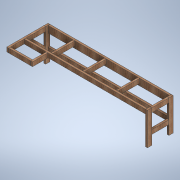
# Autodesk Inventor part: Frame Single
Saved by Autodesk Inventor 2020.2 (Build 242310000, 310)
## iProperties
Created: 2019-12-30
Part Number: Frame Single
Material: Wood (Birch - Stained)
Document SubType Name: Modeling
Designer: Andrew
Density: 0.1 g/cm^3
Appearance: Birch - Stained
Author: Andrew
Autodesk Inventor part; units mm, degrees
ref_plane "YZ Plane" through (0, 0, 0) normal (1, 0, 0) x (0, 1, 0)
ref_plane "XZ Plane" through (0, 0, 0) normal (0, 1, 0) x (-1, 0, 0)
ref_plane "XY Plane" through (0, 0, 0) normal (0, 0, 1) x (1, 0, 0)
derived "Desk Top Primary.ipt"
sketch "Primary Top" plane through (0, 0, 0) normal (0, 1, 0) x (-1, 0, 0)
  line L0 (-2713.228, 0) -> (-579.628, 0)
  line L1 (-579.628, 0) -> (-579.628, 143.3195)
  line L2 (-579.628, 143.3195) -> (-2713.228, 143.3195)
  line L3 (-2713.228, 143.3195) -> (-2713.228, 0)
  line L4 (-2713.228, 144.907) -> (-579.628, 144.907)
  line L5 (-579.628, 144.907) -> (-579.628, 288.2265)
  line L6 (-579.628, 288.2265) -> (-2713.228, 288.2265)
  line L7 (-2713.228, 288.2265) -> (-2713.228, 144.907)
  line L8 (-2713.228, 289.814) -> (-579.628, 289.814)
  line L9 (-579.628, 289.814) -> (-579.628, 433.1335)
  line L10 (-579.628, 433.1335) -> (-2713.228, 433.1335)
  line L11 (-2713.228, 433.1335) -> (-2713.228, 289.814)
  line L12 (-2713.228, 434.721) -> (-579.628, 434.721)
  line L13 (-579.628, 434.721) -> (-579.628, 578.0405)
  line L14 (-579.628, 578.0405) -> (-2713.228, 578.0405)
  line L15 (-2713.228, 578.0405) -> (-2713.228, 434.721)
  point P0 (0, 0)
derived "Desk Top Secondary.ipt"
sketch "Secondary Top" plane through (0, 0, 0) normal (0, 1, 0) x (-1, 0, 0)
  line L0 (0, 1270) -> (-143.3195, 1270)
  line L1 (-143.3195, 1270) -> (-143.3195, 0)
  line L2 (-143.3195, 0) -> (0, 0)
  line L3 (0, 0) -> (0, 1270)
  line L4 (-144.907, 1270) -> (-288.2265, 1270)
  line L5 (-288.2265, 1270) -> (-288.2265, 0)
  line L6 (-288.2265, 0) -> (-144.907, 0)
  line L7 (-144.907, 0) -> (-144.907, 1270)
  line L8 (-289.814, 1270) -> (-433.1335, 1270)
  line L9 (-433.1335, 1270) -> (-433.1335, 0)
  line L10 (-433.1335, 0) -> (-289.814, 0)
  line L11 (-289.814, 0) -> (-289.814, 1270)
  line L12 (-434.721, 1270) -> (-578.0405, 1270)
  line L13 (-578.0405, 1270) -> (-578.0405, 0)
  line L14 (-578.0405, 0) -> (-434.721, 0)
  line L15 (-434.721, 0) -> (-434.721, 1270)
sketch "Sketch3" plane through (0, 0, 0) normal (0, 1, 0) x (-1, 0, 0)
  line L0 (-12.7, 898.525) -> (-52.3966, 898.525)
  line L1 (-52.3966, 898.525) -> (-52.3966, 105.3465)
  line L2 (-52.3966, 105.3465) -> (-12.7, 105.3465)
  line L3 (-12.7, 105.3465) -> (-12.7, 898.525)
  line L4 (-12.7, 103.759) -> (-52.3966, 103.759)
  line L5 (-52.3966, 103.759) -> (-52.3966, 12.7)
  line L6 (-52.3966, 12.7) -> (-12.7, 12.7)
  line L7 (-12.7, 12.7) -> (-12.7, 103.759)
  line L8 (-53.9841, 12.7) -> (-2659.2439, 12.7)
  line L9 (-2659.2439, 12.7) -> (-2659.2439, 52.3966)
  line L10 (-2659.2439, 52.3966) -> (-53.9841, 52.3966)
  line L11 (-53.9841, 52.3966) -> (-53.9841, 12.7)
  line L12 (-2700.528, 12.7) -> (-2660.8314, 12.7)
  line L13 (-2660.8314, 12.7) -> (-2660.8314, 103.759)
  line L14 (-2660.8314, 103.759) -> (-2700.528, 103.759)
  line L15 (-2700.528, 103.759) -> (-2700.528, 12.7)
  line L16 (-2700.528, 105.3465) -> (-2660.8314, 105.3465)
  line L17 (-2660.8314, 105.3465) -> (-2660.8314, 472.694)
  line L18 (-2660.8314, 472.694) -> (-2700.528, 472.694)
  line L19 (-2700.528, 472.694) -> (-2700.528, 105.3465)
  line L20 (-2700.528, 474.2815) -> (-2660.8314, 474.2815)
  line L21 (-2660.8314, 474.2815) -> (-2660.8314, 565.3405)
  line L22 (-2660.8314, 565.3405) -> (-2700.528, 565.3405)
  line L23 (-2700.528, 565.3405) -> (-2700.528, 474.2815)
  line L24 (-2659.2439, 565.3405) -> (-53.9841, 565.3405)
  line L25 (-53.9841, 565.3405) -> (-53.9841, 525.6439)
  line L26 (-53.9841, 525.6439) -> (-2659.2439, 525.6439)
  line L27 (-2659.2439, 525.6439) -> (-2659.2439, 565.3405)
  line L28 (-53.9841, 898.525) -> (-524.0564, 898.525)
  line L29 (-524.0564, 898.525) -> (-524.0564, 858.8284)
  line L30 (-524.0564, 858.8284) -> (-53.9841, 858.8284)
  line L31 (-53.9841, 858.8284) -> (-53.9841, 898.525)
  line L32 (-565.3405, 898.525) -> (-525.6439, 898.525)
  line L33 (-525.6439, 898.525) -> (-525.6439, 566.928)
  line L34 (-525.6439, 566.928) -> (-565.3405, 566.928)
  line L35 (-565.3405, 566.928) -> (-565.3405, 898.525)
  line L36 (-2025.8314, 524.0564) -> (-1986.1349, 524.0564)
  line L37 (-1986.1349, 524.0564) -> (-1986.1349, 53.9841)
  line L38 (-1986.1349, 53.9841) -> (-2025.8314, 53.9841)
  line L39 (-2025.8314, 53.9841) -> (-2025.8314, 524.0564)
  line L40 (-592.328, 524.0564) -> (-632.0246, 524.0564)
  line L41 (-632.0246, 524.0564) -> (-632.0246, 53.9841)
  line L42 (-632.0246, 53.9841) -> (-592.328, 53.9841)
  line L43 (-592.328, 53.9841) -> (-592.328, 524.0564)
  line L44 (-1267.0246, 524.0564) -> (-1306.7211, 524.0564)
  line L45 (-1306.7211, 524.0564) -> (-1306.7211, 53.9841)
  line L46 (-1306.7211, 53.9841) -> (-1267.0246, 53.9841)
  line L47 (-1267.0246, 53.9841) -> (-1267.0246, 524.0564)
  point P0 (0, 0)
  point P1 (-2713.228, 578.0405)
  point P2 (-578.0405, 1270)
  point P3 (-579.628, 0)
  dimension "d2" = 39.6966
  dimension "d3" = 39.6966
  dimension "d4" = 39.6966
  dimension "d5" = 91.059
  dimension "d6" = 39.6966
  dimension "d7" = 39.6966
  dimension "d8" = 39.6966
  dimension "d10" = 39.6966
  dimension "d11" = 39.6966
  dimension "d12" = 91.059
  dimension "d13" = 91.059
  dimension "d14" = 39.6966
  dimension "d15" = 12.7
  dimension "d16" = 12.7
  dimension "d17" = 1.5875
  dimension "d18" = 1.5875
  dimension "d19" = 1.5875
  dimension "d20" = 1.5875
  dimension "d21" = 1.5875
  dimension "d22" = 1.5875
  dimension "d23" = 12.7
  dimension "d24" = 12.7
  dimension "d25" = 1.5875
  dimension "d26" = 1.5875
  dimension "d27" = 1.5875
  dimension "d28" = 1.5875
  dimension "d29" = 1.5875
  dimension "d30" = 1.5875
  dimension "d31" = 12.7
  dimension "d32" = 635
  dimension "d33" = 635
  dimension "d34" = 12.7
  dimension "d35" = 371.475
  dimension "d47" = 39.6966
  constraints: 96 end point, 24 parallel, 12 horizontal, 12 perpendicular, 11 point on line, 1 collinear
  measures "d2" distance of L0.start L0.end
  measures "d3" distance of L30.end L28.start
  measures "d4" distance of L32.start L32.end
  measures "d5" distance of L6.end L4.start
  measures "d6" distance of L24.end L25.end
  measures "d7" distance of L41.end L42.end
  measures "d8" distance of L45.end L46.end
  measures "d10" distance of L37.end L38.end
  measures "d11" distance of L12.start L12.end
  measures "d12" distance of L14.end L12.start
  measures "d13" distance of L22.end L20.start
  measures "d14" distance of L5.end L6.end
  measures "d15" horizontal distance of point (-2713.228, 578.041) L22.end
  measures "d16" horizontal distance of point (-2713.228, 578.041) L22.end
  measures "d17" distance between parallel lines of L21 L27
  measures "d18" distance between parallel lines of L18 L20
  measures "d19" distance between parallel lines of L14 L16
  measures "d20" distance between parallel lines of L13 L9
  measures "d21" distance between parallel lines of L11 L5
  measures "d22" distance between parallel lines of L2 L4
  measures "d23" horizontal distance of L6.end point (0, 0)
  measures "d24" horizontal distance of L6.end point (0, 0)
  measures "d25" distance between parallel lines of L10 L42
  measures "d26" distance between parallel lines of L26 L40
  measures "d27" distance between parallel lines of L24 L34
  measures "d28" distance between parallel lines of L33 L29
  measures "d29" distance between parallel lines of L31 L1
  measures "d30" distance between parallel lines of L25 L1
  measures "d31" horizontal distance of point (-578.041, 1270) L32.start
  measures "d32" distance between parallel lines of L47 L41
  measures "d33" distance between parallel lines of L17 L39
  measures "d34" distance from line of L43 point (-579.628, 0)
  measures "d35" vertical distance of point (-578.041, 1270) L32.start
  measures "d47" distance of L10.end L8.start
derived "Desk Drawer.ipt"
extrude "Extrusion1" add sketch "Sketch3" against normal blind 91.059 contours L3 L2 L1 L0 | L19 L18 L17 L16 | L24 L25 L26 L27 | L31 L30 L29 L28 | L32 L33 L34 L35 | L36 L37 L38 L39 | L43 L42 L41 L40 | L47 L46 L45 L44
extrude "Extrusion2" add sketch "Sketch3" against normal blind 698.5 contours L7 L6 L5 L4 | L15 L14 L13 L12 | L23 L22 L21 L20
derived "Frame Primary.ipt"
ref_plane "Support Plane" through (0, -495.3, 0) normal (0, 1, 0) x (-1, 0, 0)
extrude "Extrusion3" add sketch "Sketch3" along normal blind 91.059 from surface at -495.3 contours L8 L9 L10 L11 | L19 L18 L17 L16
extrude "Extrusion4" add sketch "Sketch3" against normal blind 143.3195 contours L8 L9 L10 L11
sketch "Sketch4" plane through (12.7, 0, 12.7) normal (-1, 0, 0) x (0, 0, 1)
  line L0 (366.5231, -92.6465) -> (92.6465, -366.5231)
  line L1 (92.6465, -366.5231) -> (92.6465, -495.3)
  line L2 (92.6465, -495.3) -> (495.3, -92.6465)
  line L3 (495.3, -92.6465) -> (366.5231, -92.6465)
  line L4 (91.059, 0) -> (91.059, -698.5) projected
  line L5 (885.825, -91.059) -> (92.6465, -91.059) projected
  point P0 (-12.7, 0)
  dimension "d48" = 1.5875
  dimension "d49" = 1.5875
  dimension "d50" = 91.059
  dimension "d51" = 45
  dimension "d52" = 203.2
  constraints: 8 end point, 1 parallel, 1 perpendicular, 1 vertical
  measures "d48" distance between parallel lines of L4 L1
  measures "d49" distance between parallel lines of L3 L5
  measures "d50" distance between parallel lines of L2 L0
  measures "d51" angle of L4 L0
  measures "d52" vertical distance of L4.end L1.end
extrude "Extrusion5" add sketch "Sketch4" against normal blind 39.6966
equation "\"d2\" = h_2x4"
equation "\"d3\" = h_2x4"
equation "\"d4\" = h_2x4"
equation "\"d5\" = w_2x4"
equation "\"d6\" = h_2x4"
equation "\"d7\" = h_2x4"
equation "\"d8\" = h_2x4"
equation "\"d10\" = h_2x4"
equation "\"d11\" = h_2x4"
equation "\"d12\" = w_2x4"
equation "\"d13\" = w_2x4"
equation "\"d14\" = h_2x4"
equation "\"d16\" = d15"
equation "\"d17\" = plank_tol"
equation "\"d18\" = plank_tol"
equation "\"d19\" = plank_tol"
equation "\"d20\" = plank_tol"
equation "\"d21\" = plank_tol"
equation "\"d22\" = plank_tol"
equation "\"d23\" = d15"
equation "\"d24\" = d15"
equation "\"d25\" = plank_tol"
equation "\"d26\" = plank_tol"
equation "\"d27\" = plank_tol"
equation "\"d28\" = plank_tol"
equation "\"d29\" = plank_tol"
equation "\"d30\" = plank_tol"
equation "\"d31\" = d15"
equation "\"d34\" = d15"
equation "\"d47\" = h_2x4"
equation "\"d37\" = w_2x4"
equation "\"d39\" = drawer_height"
equation "\"d42\" = w_2x4"
equation "\"d45\" = w_2x6"
equation "\"d48\" = plank_tol"
equation "\"d49\" = plank_tol"
equation "\"d50\" = w_2x4"
equation "\"d53\" = h_2x4"
equation "\"h_2x4\" = 39.696571"
equation "\"w_2x4\" = 91.059"
equation "\"plank_tol\" = 1.5875"
equation "\"drawer_height\" = 698.5"
equation "\"w_2x6\" = 143.3195"
body "Solid1"
